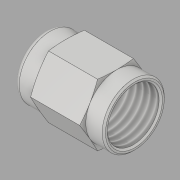
# Autodesk Inventor part: AN818-2D
Saved by Autodesk Inventor 2019 (Build 230136000, 136)
## iProperties
Created: 2018-11-23
Part Number: AN818-2D
Material: Aluminum 2014-T6
Document SubType Name: Modeling
Designer: erics
Density: 2.78927 g/cm^3
Appearance: Satin
Mass: 1.17207 g
Surface Area: 8.54531 cm^2
Volume: 0.420207 cm^3
Author: erics
Autodesk Inventor part; units mm, degrees
ref_plane "YZ Plane" through (0, 0, 0) normal (1, 0, 0) x (0, 1, 0)
ref_plane "XZ Plane" through (0, 0, 0) normal (0, 1, 0) x (-1, 0, 0)
sketch "Sketch1" plane through (0, 0, 0) normal (0, 0, 1) x (1, 0, 0)
  line L0 (0.7874, -4.7625) -> (13.5128, -4.7625)
  line L1 (13.7668, -4.5085) -> (13.7668, -4.2227)
  line L2 (13.5128, -3.9688) -> (2.3368, -3.9688)
  line L3 (2.0828, -3.7148) -> (2.0828, -2.413)
  line L4 (1.9558, -2.286) -> (0.127, -2.286)
  line L5 (0, -3.9751) -> (0, -2.413)
  arc A0 (0, -3.9751) -> (0.7874, -4.7625) centre (0.7874, -3.9751) ccw
  line L6 (0.127, -2.286) -> (0, -2.413)
  line L7 (1.9558, -2.286) -> (2.0828, -2.413)
  line L8 (13.5128, -4.7625) -> (13.7668, -4.5085)
  line L9 (13.5128, -3.9688) -> (13.7668, -4.2227)
  arc A1 (2.0828, -3.7148) -> (2.3368, -3.9688) centre (2.3368, -3.7148) ccw
  line L10 (-3.9746, 0) -> (22.117, 0) projected
  point P0 (0, 0)
  point P1 (0, -4.7625)
  point P2 (13.7668, -4.7625)
  point P3 (13.7668, -3.9688)
  point P4 (2.0828, -3.9688)
  point P5 (2.0828, -2.286)
  point P6 (0, -2.286)
  dimension "d0" = 2.286
  dimension "d1" = 4.7625
  dimension "d2" = 13.7668
  dimension "d3" = 11.684
  dimension "d4" = 0.7874
  dimension "d5" = 0.127
  dimension "d6" = 0.127
  dimension "d7" = 0.127
  dimension "d8" = 0.127
  dimension "d9" = 0.254
  dimension "d10" = 0.254
  dimension "d11" = 0.254
  dimension "d12" = 0.254
  dimension "d13" = 0.254
  dimension "d14" = 3.9688
  constraints: 20 end point, 12 point on line, 4 perpendicular, 4 point on circle, 4 tangent, 2 centre point, 2 vertical alignment, 1 horizontal, 1 vertical
  measures "d0" distance from line of point (0, 0) L4
  measures "d1" distance from line of point (0, 0) L0
  measures "d2" distance of point (0, -4.762) point (13.767, -4.762)
  measures "d3" distance of point (13.767, -3.969) point (2.083, -3.969)
  measures "d4" radius of A0
  measures "d5" distance of L4.end point (0, -2.286)
  measures "d6" distance of L5.end point (0, -2.286)
  measures "d7" distance of L4.start point (2.083, -2.286)
  measures "d8" distance of L3.end point (2.083, -2.286)
  measures "d9" distance of L0.end point (13.767, -4.762)
  measures "d10" distance of L1.start point (13.767, -4.762)
  measures "d11" distance of L2.start point (13.767, -3.969)
  measures "d12" distance of L1.end point (13.767, -3.969)
  measures "d13" radius of A1
  measures "d14" distance from line of point (0, 0) L2
revolve "Revolution1" add sketch "Sketch1" angle 360 about axis through (-10, 0, 0) along (1, 0, 0)
ref_plane "Work Plane1" through (10.9982, 0, 0) normal (1, 0, 0) x (0, 0, -1)
sketch "Sketch2" plane through (10.9982, 0, 0) normal (1, 0, 0) x (0, 0, -1)
  circle A0 centre (0, 0) radius 3.9688 projected
  circle A1 centre (0, 0) radius 4.7625 projected
  line L0 (2.7496, 4.7625) -> (5.4993, 0)
  line L1 (5.4993, 0) -> (2.7496, -4.7625)
  line L2 (2.7496, -4.7625) -> (-2.7496, -4.7625)
  line L3 (-2.7496, -4.7625) -> (-5.4993, 0)
  line L4 (-5.4993, 0) -> (-2.7496, 4.7625)
  line L5 (-2.7496, 4.7625) -> (2.7496, 4.7625)
  dimension "d24" = 9.525
  constraints: 12 end point, 1 coincident, 1 horizontal, 13 other
  measures "d24" distance between parallel lines of L2 L5
extrude "Extrusion1" add sketch "Sketch2" against normal blind 7.9248 contours A1 L0 L1 | A1 L5 L0 | L1 L2 A1 | A1 L4 L5 | L2 L3 A1 | A1 L3 L4
sketch "Sketch3" plane through (0, 0, 0) normal (0, 1, 0) x (-1, 0, 0)
  line L0 (-13.5128, 4.7625) -> (-10.9982, 4.7625) construction
  line L1 (-10.9982, 2.7496) -> (-10.9982, 5.4993) construction
  line L2 (-3.0734, 2.7496) -> (-3.0734, 4.1244) construction
  line L3 (-10.9982, 2.7496) -> (-3.0734, 2.7496) construction
  line L4 (-10.9982, 2.7496) -> (-10.9982, 4.1244) construction
  line L5 (-10.9982, 5.4993) -> (-3.0734, 5.4993) construction
  line L6 (-3.0734, 4.7625) -> (-0.7874, 4.7625) construction
  line L7 (-10.9982, 4.7625) -> (-10.8008, 5.4993)
  line L8 (-3.0734, 4.7625) -> (-3.2708, 5.4993)
  line L9 (6.6142, 0) -> (-39.685, 0) projected
  line L10 (-3.0734, 4.7625) -> (-3.0734, 5.4993)
  line L11 (-3.2708, 5.4993) -> (-3.0734, 5.4993)
  line L12 (-10.8008, 5.4993) -> (-10.9982, 5.4993)
  line L13 (-10.9982, 4.7625) -> (-10.9982, 5.4993)
  line L14 (-10.9982, 4.1244) -> (-10.9982, 5.4993) projected
  line L15 (-3.0734, 4.1244) -> (-3.0734, 5.4993) projected
  point P0 (0, 0)
  dimension "d19" = 15
  dimension "d25" = 15
  constraints: 12 end point, 2 collinear, 2 point on line, 1 perpendicular, 1 vertical
  measures "d19" angle of L1 L7
  measures "d25" angle of L2 L8
revolve "Revolution2" cut sketch "Sketch3" angle 360 about axis through (-10, 0, 0) along (1, 0, 0)
thread "Thread1" size "5/16-24 UNF" class "3B" standard "ANSI Unified Screw Threads" length 9.5504
equation "\"d0\" = 0.5 * AN818_A"
equation "\"d1\" = 0.5 * AN818_C"
equation "\"d2\" = AN818_M"
equation "\"d3\" = AN818_L"
equation "\"d4\" = AN818_R"
equation "\"d5\" = AN818_U"
equation "\"d6\" = d5"
equation "\"d7\" = d5"
equation "\"d8\" = d7"
equation "\"d9\" = AN818_N"
equation "\"d10\" = d9"
equation "\"d11\" = d9"
equation "\"d12\" = d11"
equation "\"d14\" = 0.5 * AN818_T"
equation "\"d24\" = AN818_P"
equation "\"d17\" = AN818_J"
equation "\"d22\" = AN818_S"
equation "\"AN818_A\" = 4.572"
equation "\"AN818_B\" = 2.7686"
equation "\"AN818_C\" = 9.525"
equation "\"AN818_H\" = 7.9248"
equation "\"AN818_J\" = 7.9248"
equation "\"AN818_L\" = 11.684"
equation "\"AN818_M\" = 13.7668"
equation "\"AN818_N\" = 0.254"
equation "\"AN818_P\" = 9.525"
equation "\"AN818_Q\" = 6.3754"
equation "\"AN818_R\" = 0.7874"
equation "\"AN818_S\" = 9.5504"
equation "\"AN818_U\" = 0.127"
equation "\"AN818_T\" = 7.9375"
equation "\"d16\" = -AN818_B"
equation "\"Tube_OD\" = 3.175"
body "Solid1"
